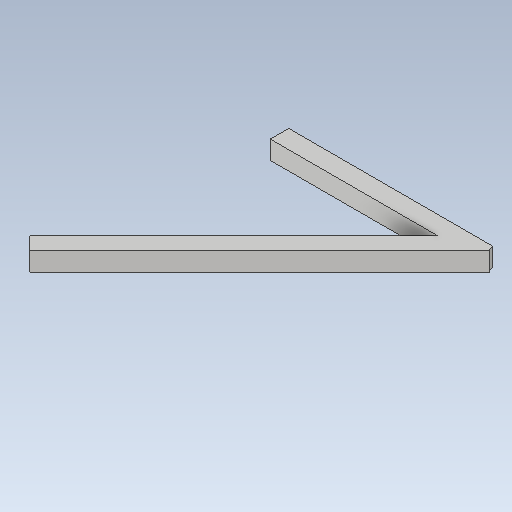
# Autodesk Inventor part: A_LeftWall2(plan)_5
Saved by Autodesk Inventor 2020 (Build 240168000, 168)
## iProperties
Created: 2020-12-21
Part Number: A_LeftWall2(plan)_5
Material: Generic
Document SubType Name: Modeling
Designer: Dell
Density: 1 g/cm^3
Appearance: Default
Author: Dell
Autodesk Inventor part; units mm, degrees
ref_plane "YZ Plane" through (0, 0, 0) normal (1, 0, 0) x (0, 1, 0)
ref_plane "XZ Plane" through (0, 0, 0) normal (0, 1, 0) x (-1, 0, 0)
ref_plane "XY Plane" through (0, 0, 0) normal (0, 0, 1) x (1, 0, 0)
sketch "Sketch1" plane through (0, 0, 0) normal (0, 1, 0) x (-1, 0, 0)
  line L0 (0, 0) -> (200, 0)
  line L1 (200, 0) -> (306.066, 106.066)
  line L2 (306.066, 106.066) -> (335.7645, 76.3675)
  line L3 (0, 0) -> (0, -42)
  line L4 (0, -42) -> (350, -42)
  line L5 (350, -42) -> (328.1362, 0)
  line L6 (350, -42) -> (414.721, -42) construction
  line L7 (261.897, 0) -> (328.1362, 0)
  line L8 (335.7645, 76.3675) -> (261.1647, 1.7678)
  arc A0 (261.1647, 1.7678) -> (261.897, 0) centre (259.397, 0) ccw
  line L9 (328.1362, 0) -> (328.1362, 6)
  line L10 (328.1362, 6) -> (273.8823, 6)
  line L11 (335.7645, 76.3675) -> (340.0071, 72.1249)
  line L12 (340.0071, 72.1249) -> (273.8823, 6)
  arc A1 (261.897, 0) -> (261.1647, 1.7678) centre (259.397, 0) ccw
  dimension "d0" = 200
  dimension "d1" = 150
  dimension "d2" = 135
  dimension "d3" = 42
  dimension "d4" = 42
  dimension "d5" = 350
  dimension "d6" = 117.5
  dimension "d8" = 5
  dimension "d9" = 6
  dimension "d10" = 6
  dimension "d13" = 66.2392
  dimension "d14" = 54.2539
  constraints: 26 end point, 6 perpendicular, 4 point on circle, 3 horizontal, 2 centre point, 2 vertical, 1 coincident, 1 point on line
  measures "d0" distance of L0.start L0.end
  measures "d1" distance of L0.end L1.end
  measures "d2" angle of L1 L0
  measures "d3" distance of L1.end L2.end
  measures "d4" distance of L0.start L3.end
  measures "d5" distance of L3.end L4.end
  measures "d6" angle of L6 L5
  measures "d8" diameter of A0
  measures "d9" distance of L5.end L9.end
  measures "d10" distance of L2.end L11.end
  measures "d13" distance of L7.start L5.end
  measures "d14" distance of L9.end L10.end
extrude "Extrusion1" add sketch "Sketch1" along normal blind 6 contours L11 L12 L10 L9 L7 A1 L8
body "Solid1"
